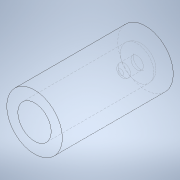
# Autodesk Inventor part: coax_test
Saved by Autodesk Inventor 2022 (Build 260153000, 153)
## iProperties
Part Number: coax_test
Material: Generic
Document SubType Name: Modeling
Designer: cssri
Appearance: Default
Author: cssri
Autodesk Inventor part; units mm, degrees
ref_plane "YZ Plane" through (0, 0, 0) normal (1, 0, 0) x (0, 1, 0)
ref_plane "XZ Plane" through (0, 0, 0) normal (0, 1, 0) x (-1, 0, 0)
ref_plane "XY Plane" through (0, 0, 0) normal (0, 0, 1) x (1, 0, 0)
sketch "Sketch1" plane through (0, 0, 50.8) normal (0, 0, 1) x (1, 0, 0)
  circle A0 centre (0, 0) radius 12.7
  constraints: 1 centre point
sketch "Sketch2" plane through (0, 0, 0) normal (0, 1, 0) x (-1, 0, 0)
  line L0 (0, 50.8) -> (-7.62, 50.8)
  line L1 (-7.62, 50.8) -> (-7.62, 3.81)
  arc A0 (-7.62, 3.81) -> (-2.8448, 3.81) centre (-5.2324, 3.81) ccw
  line L2 (-2.8448, 3.81) -> (-2.8448, 9.6774)
  arc A1 (-1.2573, 11.2649) -> (-2.8448, 9.6774) centre (-1.2573, 9.6774) ccw
  line L3 (-1.2573, 11.2649) -> (0, 11.2649)
  line L4 (0, 11.2649) -> (0, 50.8)
  line L5 (0, -10.16) -> (0, 60.96) projected
  constraints: 10 end point, 4 point on circle, 2 centre point
extrude "Extrusion1" add sketch "Sketch1" against normal blind 50.8
revolve "Revolution1" cut sketch "Sketch2" angle 360 about axis through (0, 0, -10) along (0, 0, 1)
body "Solid1"
